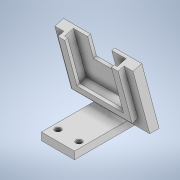
# Autodesk Inventor part: Camera_Mount
Saved by Autodesk Inventor 2022 (Build 260153000, 153)
## iProperties
Created: 2022-04-26
Part Number: Camera_Mount
Material: Generic
Document SubType Name: Modeling
Designer: Mlees
Density: 1 g/cm^3
Appearance: Default
Author: Mlees
Autodesk Inventor part; units mm, degrees
ref_plane "YZ Plane" through (0, 0, 0) normal (1, 0, 0) x (0, 1, 0)
ref_plane "XZ Plane" through (0, 0, 0) normal (0, 1, 0) x (-1, 0, 0)
ref_plane "XY Plane" through (0, 0, 0) normal (0, 0, 1) x (1, 0, 0)
sketch "Sketch1" plane through (0, 0, 0) normal (1, 0, 0) x (0, 1, 0)
  line L0 (0, 0) -> (5, 0)
  line L1 (5, 0) -> (5, -35)
  line L2 (5, -35) -> (46.5348, -23.8708)
  line L3 (47.4499, -27.2858) -> (46.5348, -23.8708)
  line L4 (47.4499, -27.2858) -> (48.0969, -29.7007)
  line L5 (48.0969, -29.7007) -> (0, -42.5882)
  line L6 (0, -42.5882) -> (0, 0)
  dimension "d0" = 5
  dimension "d1" = 35
  dimension "d2" = 43
  dimension "d3" = 75
  dimension "d5" = 2.5
  constraints: 14 end point, 2 perpendicular, 1 horizontal, 1 vertical
  measures "d0" distance of L0.start L0.end
  measures "d1" distance of L0.end L1.end
  measures "d2" distance of L1.end L2.end
  measures "d3" angle of L2 L1
  measures "d5" distance of L3.start L4.end
extrude "Extrusion1" add sketch "Sketch1" along normal blind 22
sketch "Sketch2" plane through (0, 46.5348, -23.8708) normal (0, 0.9659258, 0.258819) x (1, 0, 0)
  line L0 (0, 0) -> (22, 0) projected
  line L1 (22, -35.1015) -> (22, 6.0355) projected
  line L2 (22, 0) -> (22, 6.0355)
  line L3 (22, 3.0178) -> (0, 3.0178)
  line L4 (0, -35.1015) -> (0, 6.0355) projected
  line L5 (0, 0) -> (22, 0)
  line L6 (22, 0) -> (22, 3.0178)
  line L7 (22, 3.0178) -> (0, 3.0178)
  line L8 (0, 3.0178) -> (0, 0)
  point P0 (22, 3.0178)
  constraints: 12 end point, 2 horizontal, 2 parallel, 1 midpoint, 1 perpendicular, 1 point on line, 1 vertical
extrude "Extrusion2" cut sketch "Sketch2" against normal blind 33.404
sketch "Sketch3" plane through (22, 0, 0) normal (1, 0, 0) x (0, 0, -1)
  line L0 (35, 5) -> (41.2484, 5)
  line L1 (42.5882, 0) -> (29.7007, 48.0969) projected
  line L2 (29.7007, 48.0969) -> (26.7857, 47.3159) projected
  line L3 (41.2484, 5) -> (29.7007, 48.0969)
  line L4 (29.7007, 48.0969) -> (26.7857, 47.3159)
  line L5 (35.4313, 15.0501) -> (26.7857, 47.3159) projected
  line L6 (26.7857, 47.3159) -> (35.4313, 15.0501)
  line L7 (32.5164, 14.269) -> (35.4313, 15.0501) projected
  line L8 (35.4313, 15.0501) -> (32.5164, 14.269)
  line L9 (32.5164, 14.269) -> (35, 5) projected
  line L10 (32.5164, 14.269) -> (35, 5)
  point P0 (0, 0)
  constraints: 12 end point, 4 perpendicular, 1 collinear, 1 horizontal, 1 point on line
extrude "Extrusion3" add sketch "Sketch3" along normal blind 15
sketch "Sketch4" plane through (0, 0, 0) normal (-1, 0, 0) x (0, 0, 1)
  line L0 (-42.5882, 0) -> (-41.2484, 5) projected
  line L1 (-42.5882, 0) -> (-29.7007, 48.0969) projected
  line L2 (-42.5882, 0) -> (-29.7007, 48.0969)
  line L3 (-29.7007, 48.0969) -> (-26.7857, 47.3159) projected
  line L4 (-29.7007, 48.0969) -> (-26.7857, 47.3159)
  line L5 (-32.5164, 14.269) -> (-35.4313, 15.0501) projected
  line L6 (-26.7857, 47.3159) -> (-35.4313, 15.0501)
  line L7 (-35.4313, 15.0501) -> (-32.5164, 14.269)
  line L8 (-32.5164, 14.269) -> (-35, 5)
  line L9 (-35, 5) -> (-41.2484, 5) projected
  line L10 (-35, 5) -> (-41.2484, 5)
  point P0 (0, 0)
  constraints: 12 end point, 3 collinear, 3 perpendicular
extrude "Extrusion4" add sketch "Sketch4" along normal blind 15
sketch "Sketch5" plane through (-15, 47.3159, -26.7857) normal (0, 0.9659258, 0.258819) x (1, 0, 0)
  line L0 (0, 3.0178) -> (0, -3.0178) projected
  line L1 (0, -3.0178) -> (0, 0) projected
  line L2 (0, 3.0178) -> (0, -3.0178)
  line L3 (0, 3.0178) -> (52, 3.0178) projected
  line L4 (52, -3.0178) -> (0, -3.0178) projected
  line L5 (52, 3.0178) -> (52, -3.0178)
  line L6 (15, -3.0178) -> (37, -3.0178) projected
  line L7 (26, -3.0178) -> (8.5, -3.0178)
  line L8 (26, -3.0178) -> (43.5, -3.0178)
  line L9 (43.5, -3.0178) -> (43.5, 3.0178)
  line L10 (43.5, 3.0178) -> (52, 3.0178)
  line L11 (52, -3.0178) -> (43.5, -3.0178)
  line L12 (8.5, -3.0178) -> (8.5, 3.0178)
  line L13 (8.5, 3.0178) -> (0, 3.0178)
  line L14 (0, -3.0178) -> (8.5, -3.0178)
  point P0 (15, -38.1193)
  dimension "d14" = 17.5
  dimension "d15" = 17.5
  constraints: 20 end point, 4 point on line, 3 collinear, 3 perpendicular, 2 vertical, 1 midpoint
  measures "d14" distance of L7.start L7.end
  measures "d15" distance of L7.start L8.end
extrude "Extrusion5" add sketch "Sketch5" against normal up to surface (33.404 mm away) contours L3 L12 L4 L0 | L3 L5 L4 L9
sketch "Sketch6" plane through (22, 5, -35) normal (0, -0.258819, 0.9659258) x (1, 0, 0)
  line L0 (-28.5, 43) -> (-28.5, 9.596) projected
  line L1 (-28.5, 43) -> (-26.5, 43)
  line L2 (-28.5, 43) -> (6.5, 43) projected
  line L3 (-26.5, 43) -> (-26.5, 11.596)
  line L4 (6.5, 9.596) -> (-28.5, 9.596) projected
  line L5 (-26.5, 11.596) -> (4.5, 11.596)
  line L6 (4.5, 11.596) -> (4.5, 43)
  line L7 (6.5, 9.596) -> (6.5, 43) projected
  line L8 (4.5, 43) -> (6.5, 43)
  line L9 (6.5, 43) -> (9, 43)
  line L10 (6.5, 43) -> (15, 43) projected
  line L11 (9, 43) -> (9, 7.096)
  line L12 (9, 7.096) -> (-31, 7.096)
  line L13 (-31, 7.096) -> (-31, 43)
  line L14 (-37, 43) -> (15, 43) projected
  line L15 (-31, 43) -> (-26.5, 43)
  point P0 (-22, 4.229)
  dimension "d18" = 2
  dimension "d19" = 31.404
  dimension "d20" = 31
  dimension "d21" = 2.5
  dimension "d22" = 35.904
  dimension "d23" = 40
  constraints: 20 end point, 4 perpendicular, 4 point on line, 3 horizontal, 1 collinear
  measures "d18" distance of L0.start L1.end
  measures "d19" distance of L1.end L3.end
  measures "d20" distance of L3.end L5.end
  measures "d21" distance of L2.end L9.end
  measures "d22" distance of L9.end L11.end
  measures "d23" distance of L11.end L12.end
extrude "Extrusion6" add sketch "Sketch6" along normal blind 4 contours L1 L3 L5 L6 L2 L7 L4 L0 | L0 L4 L7 L9 L11 L12 L13 L14
sketch "Sketch7" plane through (-15, 48.0969, -29.7007) normal (0, 0.9659258, 0.258819) x (1, 0, 0)
  line L0 (8.5, -3.0178) -> (43.5, -3.0178) projected
  line L1 (0, 0) -> (52, 0) projected
  line L2 (26, -3.0178) -> (34, -3.0178)
  line L3 (34, -3.0178) -> (34, 0)
  line L4 (34, 0) -> (26, 0)
  line L5 (26, -3.0178) -> (18, -3.0178)
  line L6 (18, -3.0178) -> (18, 0)
  line L7 (18, 0) -> (26, 0)
  point P0 (15, -41.137)
  point P1 (18, -3.0178)
  point P2 (34, -3.0178)
  dimension "d26" = 8
  dimension "d27" = 8
  constraints: 12 end point, 2 horizontal, 2 parallel, 2 perpendicular, 2 point on line, 1 midpoint
  measures "d26" distance of L4.end L3.end
  measures "d27" distance of L6.end L7.end
extrude "Extrusion7" cut sketch "Sketch7" against normal blind 15
sketch "Sketch8" plane through (0, 5, 0) normal (0, 1, 0) x (1, 0, 0)
  line L0 (0, 35) -> (0, 0) projected
  line L1 (0, 35) -> (0, 7)
  line L2 (0, 0) -> (22, 0) projected
  point P0 (4, 7)
  point P1 (18, 7)
  dimension "d30" = 28
  constraints: 2 end point, 1 point on line
  measures "d30" distance of L0.start L1.end
hole "Hole1" at (4, 5, -7) at (18, 5, -7) direction (0, -1, 0) diameter 3.25 end through all countersink diameter 4 countersink angle 90
sketch "Sketch9" plane through (-6.5, 15.0501, -35.4313) normal (0, -0.258819, 0.9659258) x (1, 0, 0)
  line L0 (0, 33.404) -> (0, 0) projected
  line L1 (0, 33.404) -> (9.5, 33.404) projected
  line L2 (0, 33.404) -> (9.5, 33.404)
  line L3 (9.5, 18.404) -> (25.5, 18.404) projected
  line L4 (9.5, 33.404) -> (9.5, 18.404)
  line L5 (9.5, 18.404) -> (25.5, 18.404)
  line L6 (25.5, 33.404) -> (25.5, 18.404) projected
  line L7 (25.5, 18.404) -> (25.5, 33.404)
  line L8 (25.5, 33.404) -> (35, 33.404) projected
  line L9 (25.5, 33.404) -> (35, 33.404)
  line L10 (35, 0) -> (35, 33.404) projected
  line L11 (35, 33.404) -> (35, 0)
  line L12 (0, 0) -> (35, 0) projected
  line L13 (35, 0) -> (0, 0)
  line L14 (0, 0) -> (0, 33.404)
  point P0 (6.5, -5.367)
  constraints: 16 end point, 4 perpendicular, 3 collinear, 1 horizontal
extrude "Extrusion8" cut sketch "Sketch9" against normal blind 1
sketch "Sketch10" plane through (31, 46.5348, -23.8708) normal (0, 0.9659258, 0.258819) x (1, 0, 0)
  line L0 (-37.5, 4.0178) -> (-37.5, 0) projected
  line L1 (-37.5, 0) -> (-37.5, -2)
  line L2 (-35.5, 0) -> (-35.5, -4) projected
  line L3 (-37.5, -2) -> (-2.5, -2)
  line L4 (-2.5, 0) -> (-2.5, 4.0178) projected
  line L5 (-2.5, -2) -> (-2.5, 0)
  line L6 (-2.5, 0) -> (-37.5, 0)
  point P0 (-31, -35.1015)
  constraints: 8 end point, 3 perpendicular, 1 parallel
extrude "Extrusion9" cut sketch "Sketch10" against normal up to surface (33.404 mm away)
body "Solid1"
